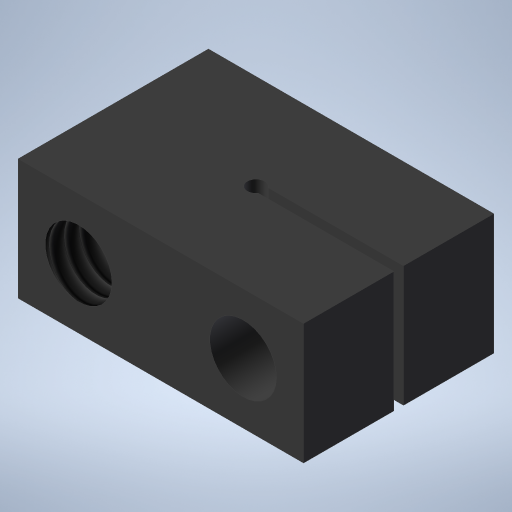
# Autodesk Inventor part: clamp(6-32)
Saved by Autodesk Inventor 2024 (Build 280153000, 153)
## iProperties
Created: 2023-04-27
Part Number: clamp(6-32)
Material: Generic
Document SubType Name: Modeling
Designer: Fujitsu
Density: 1 g/cm^3
Appearance: Default
Author: Fujitsu
Autodesk Inventor part; units mm, degrees
ref_plane "YZ Plane" through (0, 0, 0) normal (1, 0, 0) x (0, 1, 0)
ref_plane "XZ Plane" through (0, 0, 0) normal (0, 1, 0) x (-1, 0, 0)
ref_plane "XY Plane" through (0, 0, 0) normal (0, 0, 1) x (1, 0, 0)
sketch "Sketch1" plane through (0, 0, 0) normal (0, 1, 0) x (-1, 0, 0)
  line L0 (0, 0) -> (15, 0)
  line L1 (15, 0) -> (15, -10)
  line L2 (15, -10) -> (0, -10)
  line L3 (0, -10) -> (0, 0)
  line L4 (0, -5) -> (7.5006, -5)
  circle A0 centre (7.5006, -5) radius 0.4572
  line L5 (0, -5.254) -> (7.1205, -5.254)
  line L6 (0, -4.746) -> (7.1205, -4.746)
  dimension "d0" = 15
  dimension "d1" = 10
  dimension "d2" = 7.5006
  dimension "d3" = 0.9144
  dimension "d4" = 0.254
  dimension "d5" = 0.254
  constraints: 14 end point, 4 parallel, 2 horizontal, 2 point on circle, 1 centre point, 1 coincident, 1 midpoint, 1 perpendicular
  measures "d0" distance of L1.end L2.end
  measures "d1" distance of L0.end L1.end
  measures "d2" distance of L4.start L4.end
  measures "d3" diameter of A0
  measures "d4" distance between parallel lines of L4 L5
  measures "d5" distance between parallel lines of L4 L6
extrude "Extrusion1" add sketch "Sketch1" along normal blind 6.35 contours L0 L1 L2 L3 L5 A0 L6
sketch "Sketch2" plane through (-15, 0, 0) normal (0, 0, 1) x (1, 0, 0)
  line L0 (7.8795, 0) -> (15, 0) projected
  line L1 (15, 0) -> (8.65, 6.35)
  line L2 (15, 6.35) -> (7.8795, 6.35) projected
  line L3 (15, 0) -> (23.9803, 0) construction
  circle A0 centre (11.825, 3.175) radius 1.7526
  line L4 (15, 0) -> (0, 0) projected
  line L5 (0, 0) -> (6.35, 6.35)
  line L6 (7.0422, 6.35) -> (7.8795, 6.35) projected
  line L7 (0, 0) -> (8.9803, 0) construction
  circle A1 centre (3.175, 3.175) radius 1.7526
  dimension "d8" = 135
  dimension "d9" = 3.5052
  dimension "d10" = 45
  dimension "d11" = 3.5052
  constraints: 8 end point, 2 centre point, 2 equal length, 2 horizontal, 2 midpoint, 2 point on line
  measures "d8" angle of L3 L1
  measures "d9" diameter of A0
  measures "d10" angle of L7 L5
  measures "d11" diameter of A1
hole "Hole1" at (-11.825, 3.175, 0) direction (0, 0, -1) diameter 3.5052 end through all
hole "Hole2" at (-3.175, 3.175, 0) direction (0, 0, -1) diameter 3.5052 end through all
thread "Thread1" size "6-32 UNC" class "2B" standard "ANSI Unified Screw Threads" full length
thread "Thread2" size "6-32 UNC" class "2B" standard "ANSI Unified Screw Threads" full length
sketch "Sketch3" plane through (-15, 0, -10) normal (-1, 0, 0) x (0, 0, 1)
  line L0 (0, 6.35) -> (10, 6.35) projected
  line L1 (0, 6.35) -> (10, 0)
  circle A0 centre (5, 3.175) radius 0.508
  dimension "d30" = 1.016
  constraints: 2 end point, 1 centre point, 1 midpoint
  measures "d30" diameter of A0
extrude "Extrusion2" cut sketch "Sketch3" against normal blind 3.5001
body "Solid1"
